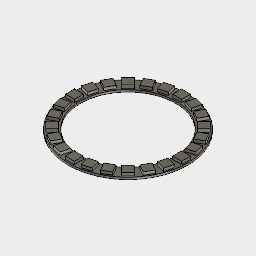
1586 24x NeoRing (Autodesk Fusion 360 design; units mm, degrees)
Autodesk Fusion 360 part; units mm, degrees
sketch "Sketch1" plane through (0, 0, 0) normal (0, 0, 1) x (1, 0, 0)
  circle A0 centre (0, 0) radius 33
  circle A1 centre (0, 0) radius 26.25
  line L0 (0.0215, 33) -> (0.0215, 26.25) construction
  line L1 (2.5215, 27.125) -> (-2.4785, 27.125)
  line L2 (-2.4785, 27.125) -> (-2.4785, 32.125)
  line L3 (-2.4785, 32.125) -> (2.5215, 32.125)
  line L4 (2.5215, 32.125) -> (2.5215, 27.125)
  line L5 (2.5215, 27.125) -> (-2.4785, 32.125) construction
  line L6 (-2.4785, 27.125) -> (2.5215, 32.125) construction
  line L7 (-10.7086, 30.3889) -> (-5.879, 31.683)
  line L8 (-5.879, 31.683) -> (-4.5849, 26.8533)
  line L9 (-4.5849, 26.8533) -> (-9.4145, 25.5592)
  line L10 (-9.4145, 25.5592) -> (-10.7086, 30.3889)
  line L11 (-18.2089, 26.5818) -> (-13.8788, 29.0818)
  line L12 (-13.8788, 29.0818) -> (-11.3788, 24.7517)
  line L13 (-11.3788, 24.7517) -> (-15.7089, 22.2517)
  line L14 (-15.7089, 22.2517) -> (-18.2089, 26.5818)
  line L15 (-24.4684, 20.9632) -> (-20.9328, 24.4988)
  line L16 (-20.9328, 24.4988) -> (-17.3973, 20.9632)
  line L17 (-17.3973, 20.9632) -> (-20.9328, 17.4277)
  line L18 (-20.9328, 17.4277) -> (-24.4684, 20.9632)
  line L19 (-29.0603, 13.9161) -> (-26.5603, 18.2462)
  line L20 (-26.5603, 18.2462) -> (-22.2302, 15.7462)
  line L21 (-22.2302, 15.7462) -> (-24.7302, 11.4161)
  line L22 (-24.7302, 11.4161) -> (-29.0603, 13.9161)
  line L23 (-31.6718, 5.9205) -> (-30.3777, 10.7501)
  line L24 (-30.3777, 10.7501) -> (-25.5481, 9.456)
  line L25 (-25.5481, 9.456) -> (-26.8422, 4.6264)
  line L26 (-26.8422, 4.6264) -> (-31.6718, 5.9205)
  line L27 (-32.125, -2.4785) -> (-32.125, 2.5215)
  line L28 (-32.125, 2.5215) -> (-27.125, 2.5215)
  line L29 (-27.125, 2.5215) -> (-27.125, -2.4785)
  line L30 (-27.125, -2.4785) -> (-32.125, -2.4785)
  line L31 (-30.3889, -10.7086) -> (-31.683, -5.879)
  line L32 (-31.683, -5.879) -> (-26.8533, -4.5849)
  line L33 (-26.8533, -4.5849) -> (-25.5592, -9.4145)
  line L34 (-25.5592, -9.4145) -> (-30.3889, -10.7086)
  line L35 (-26.5818, -18.2089) -> (-29.0818, -13.8788)
  line L36 (-29.0818, -13.8788) -> (-24.7517, -11.3788)
  line L37 (-24.7517, -11.3788) -> (-22.2517, -15.7089)
  line L38 (-22.2517, -15.7089) -> (-26.5818, -18.2089)
  line L39 (-20.9632, -24.4684) -> (-24.4988, -20.9328)
  line L40 (-24.4988, -20.9328) -> (-20.9632, -17.3973)
  line L41 (-20.9632, -17.3973) -> (-17.4277, -20.9328)
  line L42 (-17.4277, -20.9328) -> (-20.9632, -24.4684)
  line L43 (-13.9161, -29.0603) -> (-18.2462, -26.5603)
  line L44 (-18.2462, -26.5603) -> (-15.7462, -22.2302)
  line L45 (-15.7462, -22.2302) -> (-11.4161, -24.7302)
  line L46 (-11.4161, -24.7302) -> (-13.9161, -29.0603)
  line L47 (-5.9205, -31.6718) -> (-10.7501, -30.3777)
  line L48 (-10.7501, -30.3777) -> (-9.456, -25.5481)
  line L49 (-9.456, -25.5481) -> (-4.6264, -26.8422)
  line L50 (-4.6264, -26.8422) -> (-5.9205, -31.6718)
  line L51 (2.4785, -32.125) -> (-2.5215, -32.125)
  line L52 (-2.5215, -32.125) -> (-2.5215, -27.125)
  line L53 (-2.5215, -27.125) -> (2.4785, -27.125)
  line L54 (2.4785, -27.125) -> (2.4785, -32.125)
  line L55 (10.7086, -30.3889) -> (5.879, -31.683)
  line L56 (5.879, -31.683) -> (4.5849, -26.8533)
  line L57 (4.5849, -26.8533) -> (9.4145, -25.5592)
  line L58 (9.4145, -25.5592) -> (10.7086, -30.3889)
  line L59 (18.2089, -26.5818) -> (13.8788, -29.0818)
  line L60 (13.8788, -29.0818) -> (11.3788, -24.7517)
  line L61 (11.3788, -24.7517) -> (15.7089, -22.2517)
  line L62 (15.7089, -22.2517) -> (18.2089, -26.5818)
  line L63 (24.4684, -20.9632) -> (20.9328, -24.4988)
  line L64 (20.9328, -24.4988) -> (17.3973, -20.9632)
  line L65 (17.3973, -20.9632) -> (20.9328, -17.4277)
  line L66 (20.9328, -17.4277) -> (24.4684, -20.9632)
  line L67 (29.0603, -13.9161) -> (26.5603, -18.2462)
  line L68 (26.5603, -18.2462) -> (22.2302, -15.7462)
  line L69 (22.2302, -15.7462) -> (24.7302, -11.4161)
  line L70 (24.7302, -11.4161) -> (29.0603, -13.9161)
  line L71 (31.6718, -5.9205) -> (30.3777, -10.7501)
  line L72 (30.3777, -10.7501) -> (25.5481, -9.456)
  line L73 (25.5481, -9.456) -> (26.8422, -4.6264)
  line L74 (26.8422, -4.6264) -> (31.6718, -5.9205)
  line L75 (32.125, 2.4785) -> (32.125, -2.5215)
  line L76 (32.125, -2.5215) -> (27.125, -2.5215)
  line L77 (27.125, -2.5215) -> (27.125, 2.4785)
  line L78 (27.125, 2.4785) -> (32.125, 2.4785)
  line L79 (30.3889, 10.7086) -> (31.683, 5.879)
  line L80 (31.683, 5.879) -> (26.8533, 4.5849)
  line L81 (26.8533, 4.5849) -> (25.5592, 9.4145)
  line L82 (25.5592, 9.4145) -> (30.3889, 10.7086)
  line L83 (26.5818, 18.2089) -> (29.0818, 13.8788)
  line L84 (29.0818, 13.8788) -> (24.7517, 11.3788)
  line L85 (24.7517, 11.3788) -> (22.2517, 15.7089)
  line L86 (22.2517, 15.7089) -> (26.5818, 18.2089)
  line L87 (20.9632, 24.4684) -> (24.4988, 20.9328)
  line L88 (24.4988, 20.9328) -> (20.9632, 17.3973)
  line L89 (20.9632, 17.3973) -> (17.4277, 20.9328)
  line L90 (17.4277, 20.9328) -> (20.9632, 24.4684)
  line L91 (13.9161, 29.0603) -> (18.2462, 26.5603)
  line L92 (18.2462, 26.5603) -> (15.7462, 22.2302)
  line L93 (15.7462, 22.2302) -> (11.4161, 24.7302)
  line L94 (11.4161, 24.7302) -> (13.9161, 29.0603)
  line L95 (5.9205, 31.6718) -> (10.7501, 30.3777)
  line L96 (10.7501, 30.3777) -> (9.456, 25.5481)
  line L97 (9.456, 25.5481) -> (4.6264, 26.8422)
  line L98 (4.6264, 26.8422) -> (5.9205, 31.6718)
  point P0 (0.0215, 29.625)
  dimension "d1" = 66
  dimension "d2" = 52.5
  dimension "d3" = 5
  dimension "d4" = 5
  dimension "d6" = 360
  measures "d1" diameter of A0
  measures "d2" diameter of A1
  measures "d3" distance of L2.end L3.end
  measures "d4" distance of L1.end L2.end
extrude "Extrude1" add sketch "Sketch1" against normal blind 1.2 contours A0 | L1 L2 L3 L4 | L7 L8 L9 L10 | L11 L12 L13 L14 | L15 L16 L17 L18 | L19 L20 L21 L22 | L23 L24 L25 L26 | L27 L28 L29 L30 | L31 L32 L33 L34 | L35 L36 L37 L38 | L39 L40 L41 L42 | L43 L44 L45 L46 | L47 L48 L49 L50 | L51 L52 L53 L54 | L55 L56 L57 L58 | L59 L60 L61 L62 | L63 L64 L65 L66 | L67 L68 L69 L70 | L71 L72 L73 L74 | L75 L76 L77 L78 | L79 L80 L81 L82 | L83 L84 L85 L86 | L87 L88 L89 L90 | L91 L92 L93 L94 | L95 L96 L97 L98
extrude "Extrude2" add sketch "Sketch1" along normal blind 1.6 contours L1 L2 L3 L4 | L7 L8 L9 L10 | L11 L12 L13 L14 | L15 L16 L17 L18 | L19 L20 L21 L22 | L23 L24 L25 L26 | L27 L28 L29 L30 | L31 L32 L33 L34 | L35 L36 L37 L38 | L39 L40 L41 L42 | L43 L44 L45 L46 | L47 L48 L49 L50 | L51 L52 L53 L54 | L55 L56 L57 L58 | L59 L60 L61 L62 | L63 L64 L65 L66 | L67 L68 L69 L70 | L71 L72 L73 L74 | L75 L76 L77 L78 | L79 L80 L81 L82 | L83 L84 L85 L86 | L87 L88 L89 L90 | L91 L92 L93 L94 | L95 L96 L97 L98
named bodies: "24x ring"
